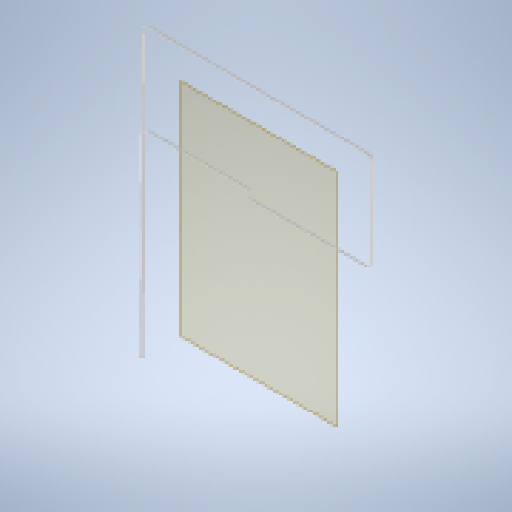
# Autodesk Inventor part: beltTest
Saved by Autodesk Inventor 2023 (Build 270158000, 158)
## iProperties
Created: 2023-08-21
Part Number: beltTest
Material: Generic
Document SubType Name: Modeling
Designer: Felix
Density: 1 g/cm^3
Appearance: Default
Author: Felix
Autodesk Inventor part; units mm, degrees
ref_plane "YZ Plane" through (0, 0, 0) normal (1, 0, 0) x (0, 1, 0)
ref_plane "XZ Plane" through (0, 0, 0) normal (0, 1, 0) x (-1, 0, 0)
ref_plane "XY Plane" through (0, 0, 0) normal (0, 0, 1) x (1, 0, 0)
ref_plane "Work Plane1" through (-397.1404, 162.2819, -117.4746) normal (0, 0, 1) x (1, 0, 0)
sketch "Sketch1" plane through (-397.1404, 162.2819, -117.4746) normal (0, 0, 1) x (1, 0, 0)
  circle A0 centre (-324.3, 142.5254) radius 11 construction
  circle A1 centre (-324.3, 410) radius 11 construction
  circle A2 centre (324.3, 410) radius 11 construction
  circle A3 centre (324.3, 142.5254) radius 11 construction
  circle A4 centre (-340.65, -430) radius 6.3842 construction
  arc A5 (-344.1203, -433.099) -> (-344.7505, -432.1984) centre (-344.419, -432.6372) ccw construction
  arc A6 (-344.9905, -432.1415) -> (-344.7505, -432.1984) centre (-344.847, -432.0707) ccw construction
  arc A7 (-345.1624, -431.7504) -> (-344.9905, -432.1415) centre (-340.65, -430) ccw construction
  arc A8 (-345.0421, -431.5351) -> (-345.1624, -431.7504) centre (-345.0132, -431.6925) ccw construction
  arc A9 (-345.0421, -431.5351) -> (-345.2797, -430.4618) centre (-345.1413, -430.9941) ccw construction
  arc A10 (-345.4796, -430.3175) -> (-345.2797, -430.4618) centre (-345.3199, -430.307) ccw construction
  arc A11 (-345.4888, -429.8903) -> (-345.4796, -430.3175) centre (-340.65, -430) ccw construction
  arc A12 (-345.2952, -429.7375) -> (-345.4888, -429.8903) centre (-345.3288, -429.8939) ccw construction
  arc A13 (-345.2952, -429.7375) -> (-345.104, -428.655) centre (-345.1799, -429.1997) ccw construction
  arc A14 (-345.2334, -428.4451) -> (-345.104, -428.655) centre (-345.0819, -428.4965) ccw construction
  arc A15 (-345.0784, -428.0469) -> (-345.2334, -428.4451) centre (-340.65, -430) ccw construction
  arc A16 (-344.8412, -427.9798) -> (-345.0784, -428.0469) centre (-344.932, -428.1115) ccw construction
  arc A17 (-344.8412, -427.9798) -> (-344.2502, -427.0529) centre (-344.5288, -427.5271) ccw construction
  arc A18 (-344.2895, -426.8095) -> (-344.2502, -427.0529) centre (-344.1692, -426.9149) ccw construction
  arc A19 (-343.9939, -426.5009) -> (-344.2895, -426.8095) centre (-340.65, -430) ccw construction
  arc A20 (-343.749, -426.5297) -> (-343.9939, -426.5009) centre (-343.8834, -426.6166) ccw construction
  arc A21 (-343.749, -426.5297) -> (-342.8484, -425.8995) centre (-343.2872, -426.231) ccw construction
  arc A22 (-342.7915, -425.6595) -> (-342.8484, -425.8995) centre (-342.7207, -425.803) ccw construction
  arc A23 (-342.4004, -425.4876) -> (-342.7915, -425.6595) centre (-340.65, -430) ccw construction
  arc A24 (-342.1851, -425.6079) -> (-342.4004, -425.4876) centre (-342.3425, -425.6368) ccw construction
  arc A25 (-342.1851, -425.6079) -> (-341.1118, -425.3703) centre (-341.6441, -425.5087) ccw construction
  arc A26 (-340.9675, -425.1704) -> (-341.1118, -425.3703) centre (-340.957, -425.3301) ccw construction
  arc A27 (-340.5403, -425.1612) -> (-340.9675, -425.1704) centre (-340.65, -430) ccw construction
  arc A28 (-340.3875, -425.3548) -> (-340.5403, -425.1612) centre (-340.5439, -425.3212) ccw construction
  arc A29 (-340.3875, -425.3548) -> (-339.305, -425.546) centre (-339.8497, -425.4701) ccw construction
  arc A30 (-339.0951, -425.4166) -> (-339.305, -425.546) centre (-339.1465, -425.5681) ccw construction
  arc A31 (-338.6969, -425.5716) -> (-339.0951, -425.4166) centre (-340.65, -430) ccw construction
  arc A32 (-338.6298, -425.8088) -> (-338.6969, -425.5716) centre (-338.7615, -425.718) ccw construction
  arc A33 (-338.6298, -425.8088) -> (-337.7029, -426.3998) centre (-338.1771, -426.1212) ccw construction
  arc A34 (-337.4595, -426.3605) -> (-337.7029, -426.3998) centre (-337.5649, -426.4808) ccw construction
  arc A35 (-337.1509, -426.6561) -> (-337.4595, -426.3605) centre (-340.65, -430) ccw construction
  arc A36 (-337.1797, -426.901) -> (-337.1509, -426.6561) centre (-337.2666, -426.7666) ccw construction
  arc A37 (-337.1797, -426.901) -> (-336.5495, -427.8016) centre (-336.881, -427.3628) ccw construction
  arc A38 (-336.3095, -427.8585) -> (-336.5495, -427.8016) centre (-336.453, -427.9293) ccw construction
  arc A39 (-336.1376, -428.2496) -> (-336.3095, -427.8585) centre (-340.65, -430) ccw construction
  arc A40 (-336.2579, -428.4649) -> (-336.1376, -428.2496) centre (-336.2868, -428.3075) ccw construction
  arc A41 (-336.2579, -428.4649) -> (-336.0203, -429.5382) centre (-336.1587, -429.0059) ccw construction
  arc A42 (-335.8204, -429.6825) -> (-336.0203, -429.5382) centre (-335.9801, -429.693) ccw construction
  arc A43 (-335.8112, -430.1097) -> (-335.8204, -429.6825) centre (-340.65, -430) ccw construction
  arc A44 (-336.0048, -430.2625) -> (-335.8112, -430.1097) centre (-335.9712, -430.1061) ccw construction
  arc A45 (-336.0048, -430.2625) -> (-336.196, -431.345) centre (-336.1201, -430.8003) ccw construction
  arc A46 (-336.0666, -431.5549) -> (-336.196, -431.345) centre (-336.2181, -431.5035) ccw construction
  arc A47 (-336.2216, -431.9531) -> (-336.0666, -431.5549) centre (-340.65, -430) ccw construction
  arc A48 (-336.4588, -432.0202) -> (-336.2216, -431.9531) centre (-336.368, -431.8885) ccw construction
  arc A49 (-336.4588, -432.0202) -> (-337.0498, -432.9471) centre (-336.7712, -432.4729) ccw construction
  arc A50 (-337.0105, -433.1905) -> (-337.0498, -432.9471) centre (-337.1308, -433.0851) ccw construction
  arc A51 (-337.3061, -433.4991) -> (-337.0105, -433.1905) centre (-340.65, -430) ccw construction
  arc A52 (-337.551, -433.4703) -> (-337.3061, -433.4991) centre (-337.4166, -433.3834) ccw construction
  arc A53 (-337.551, -433.4703) -> (-338.4516, -434.1005) centre (-338.0128, -433.769) ccw construction
  arc A54 (-338.5085, -434.3405) -> (-338.4516, -434.1005) centre (-338.5793, -434.197) ccw construction
  arc A55 (-338.8996, -434.5124) -> (-338.5085, -434.3405) centre (-340.65, -430) ccw construction
  arc A56 (-339.1149, -434.3921) -> (-338.8996, -434.5124) centre (-338.9575, -434.3632) ccw construction
  arc A57 (-339.1149, -434.3921) -> (-340.1882, -434.6297) centre (-339.6559, -434.4913) ccw construction
  arc A58 (-340.3325, -434.8296) -> (-340.1882, -434.6297) centre (-340.343, -434.6699) ccw construction
  arc A59 (-340.7597, -434.8388) -> (-340.3325, -434.8296) centre (-340.65, -430) ccw construction
  arc A60 (-340.9125, -434.6452) -> (-340.7597, -434.8388) centre (-340.7561, -434.6788) ccw construction
  arc A61 (-340.9125, -434.6452) -> (-341.995, -434.454) centre (-341.4503, -434.5299) ccw construction
  arc A62 (-342.2049, -434.5834) -> (-341.995, -434.454) centre (-342.1535, -434.4319) ccw construction
  arc A63 (-342.6031, -434.4284) -> (-342.2049, -434.5834) centre (-340.65, -430) ccw construction
  arc A64 (-342.6702, -434.1912) -> (-342.6031, -434.4284) centre (-342.5385, -434.282) ccw construction
  arc A65 (-342.6702, -434.1912) -> (-343.5971, -433.6002) centre (-343.1229, -433.8788) ccw construction
  arc A66 (-343.8405, -433.6395) -> (-343.5971, -433.6002) centre (-343.7351, -433.5192) ccw construction
  arc A67 (-344.1491, -433.3439) -> (-343.8405, -433.6395) centre (-340.65, -430) ccw construction
  arc A68 (-344.1203, -433.099) -> (-344.1491, -433.3439) centre (-344.0334, -433.2334) ccw construction
  arc A69 (-344.5998, -429.9563) -> (-336.7, -430) centre (-340.65, -430) ccw
  line L0 (-344.5998, -429.9563) -> (-335.2993, 410.1218)
  line L1 (-324.3, 421) -> (324.3, 421)
  line L2 (335.3, 410) -> (335.3, 142.5254)
  line L3 (324.3, 131.5254) -> (-24.9217, 131.5254)
  arc A70 (-324.3, 421) -> (-335.2993, 410.1218) centre (-324.3, 410) ccw
  arc A71 (324.3, 131.5254) -> (335.3, 142.5254) centre (324.3, 142.5254) ccw
  circle A72 centre (-324.3, 142.5254) radius 12.4 construction
  line L4 (-324.3, 154.9254) -> (-24.9217, 154.9254)
  line L5 (-336.7, 142.5254) -> (-336.7, -430)
  arc A73 (335.3, 410) -> (324.3, 421) centre (324.3, 410) ccw
  arc A74 (-324.3, 154.9254) -> (-336.7, 142.5254) centre (-324.3, 142.5254) ccw
  line L6 (-24.9217, 153.5254) -> (-324.3, 153.5254)
  arc A75 (-324.3, 153.5254) -> (-335.3, 142.5254) centre (-324.3, 142.5254) ccw
  line L7 (-335.3, 142.5254) -> (-335.3, -430)
  arc A76 (-345.9997, -429.9408) -> (-335.3, -430) centre (-340.65, -430) ccw
  line L8 (-345.9997, -429.9408) -> (-336.6992, 410.1373)
  arc A77 (-324.3, 422.4) -> (-336.6992, 410.1373) centre (-324.3, 410) ccw
  line L9 (-324.3, 422.4) -> (324.3, 422.4)
  arc A78 (336.7, 410) -> (324.3, 422.4) centre (324.3, 410) ccw
  line L10 (336.7, 410) -> (336.7, 142.5254)
  arc A79 (324.3, 130.1254) -> (336.7, 142.5254) centre (324.3, 142.5254) ccw
  line L11 (324.3, 130.1254) -> (-24.9217, 130.1254)
  line L12 (-24.9217, 154.9254) -> (-24.9217, 153.5254)
  line L13 (-24.9217, 131.5254) -> (-24.9217, 130.1254)
  point P0 (397.1404, -162.2819)
  dimension "d0" = 1.4
  dimension "d1" = 1.4
  constraints: 28 end point, 28 point on circle, 13 tangent, 11 centre point, 3 concentric, 2 coincident, 2 horizontal, 2 vertical, 1 collinear, 1 vertical alignment, 10 other
  measures "d0" radial gap between concentric circles of A72 A0
  measures "d1" distance between parallel lines of L4 L6
extrude "Extrusion1" add sketch "Sketch1" along normal blind 6
equation "\"d1\" = d0"
body "Solid1"
